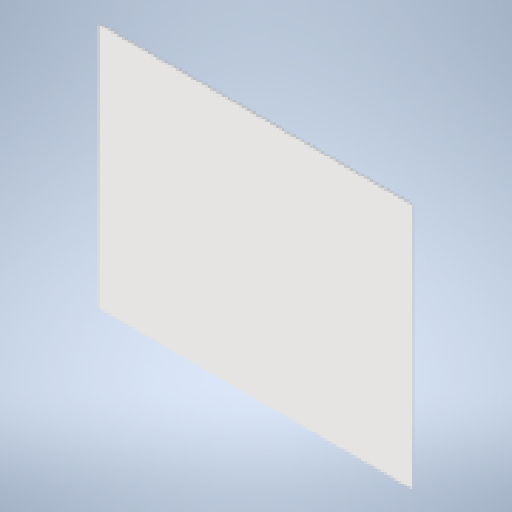
# Autodesk Inventor part: DF1.03 Wall bottom
Saved by Autodesk Inventor 2023.1 (Build 271208000, 208)
## iProperties
Created: 2023-08-31
Part Number: DF1.03 Wall bottom
Material: Generic
Document SubType Name: Modeling
Designer: admin
Density: 1 g/cm^3
Appearance: Default
Author: admin
Autodesk Inventor part; units mm, degrees
ref_plane "YZ Plane" through (0, 0, 0) normal (1, 0, 0) x (0, 1, 0)
ref_plane "XZ Plane" through (0, 0, 0) normal (0, 1, 0) x (-1, 0, 0)
ref_plane "XY Plane" through (0, 0, 0) normal (0, 0, 1) x (1, 0, 0)
sketch "Sketch1" plane through (0, 0, 0) normal (0, 0, 1) x (1, 0, 0)
  line L0 (-1100, 862.5) -> (1100, 862.5)
  line L1 (1100, 862.5) -> (1100, -862.5)
  line L2 (1100, -862.5) -> (-1100, -862.5)
  line L3 (-1100, -862.5) -> (-1100, 862.5)
  line L4 (-1100, 862.5) -> (1100, -862.5) construction
  line L5 (1100, 862.5) -> (-1100, -862.5) construction
  point P0 (0, 0)
  dimension "d0" = 1725
  dimension "d1" = 2200
  constraints: 12 end point, 2 midpoint, 2 parallel, 1 horizontal, 1 perpendicular
  measures "d0" distance of L2.end L0.start
  measures "d1" distance of L1.end L2.end
extrude "Extrusion1" add sketch "Sketch1" along normal blind 10
body "Solid1"
